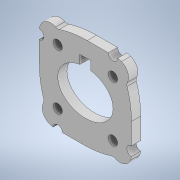
# Autodesk Inventor part: Część18
Saved by Autodesk Inventor 2021 (Build 250183000, 183)
## iProperties
Created: 2023-10-30
Part Number: Część18
Material: Ogólny
Document SubType Name: Modeling
Designer: Jakub
Density: 1 g/cm^3
Appearance: Domyślna
Author: Jakub
Autodesk Inventor part; units mm, degrees
ref_plane "YZ Plane" through (0, 0, 0) normal (1, 0, 0) x (0, 1, 0)
ref_plane "XZ Plane" through (0, 0, 0) normal (0, 1, 0) x (-1, 0, 0)
ref_plane "XY Plane" through (0, 0, 0) normal (0, 0, 1) x (1, 0, 0)
sketch "Szkic1" plane through (0, 0, 0) normal (0, 0, 1) x (1, 0, 0)
  line L0 (0, 0) -> (25, 0)
  line L1 (25, 0) -> (25, 16.5)
  line L2 (16.5, 25) -> (0, 25)
  line L3 (0, 25) -> (0, 0)
  line L4 (0, 0) -> (-25, 0)
  line L5 (-25, 0) -> (-25, -16.5)
  line L6 (-16.5, -25) -> (0, -25)
  line L7 (0, -25) -> (0, 0)
  line L8 (0, 0) -> (-25, 0)
  line L9 (-25, 0) -> (-25, 16.5)
  line L10 (-16.5, 25) -> (0, 25)
  line L11 (0, 25) -> (0, 0)
  line L12 (0, 0) -> (25, 0)
  line L13 (25, 0) -> (25, -16.5)
  line L14 (16.5, -25) -> (0, -25)
  line L15 (0, -25) -> (0, 0)
  line L16 (0, 0) -> (0, -12)
  line L17 (0, -12) -> (0, 0)
  line L18 (0, 0) -> (-15, 0)
  line L19 (-15, 0) -> (15, 0)
  line L20 (15, 0) -> (15, 12)
  line L21 (15, 12) -> (-15, 12)
  line L22 (-15, 12) -> (-15, -0.7896)
  line L23 (-15, -0.7896) -> (-15, -12)
  line L24 (-15, -12) -> (0, -12)
  line L25 (15, -12) -> (15, 0)
  line L26 (15, -12) -> (0, -12)
  ellipse E0 centre (0, 0) end of major axis (-15, 0) minor radius 12
  line L27 (0, 0) -> (0, 16.5)
  line L28 (0, 16.5) -> (3, 16.5)
  line L29 (3, 16.5) -> (3, 11.7576)
  line L30 (0, 16.5) -> (-3, 16.5)
  line L31 (-3, 16.5) -> (-3, 11.7576)
  arc A0 (-16.5, 25) -> (-25, 16.5) centre (-16.5, 16.5) ccw
  arc A1 (25, 16.5) -> (16.5, 25) centre (16.5, 16.5) ccw
  arc A2 (16.5, -25) -> (25, -16.5) centre (16.5, -16.5) ccw
  arc A3 (-25, -16.5) -> (-16.5, -25) centre (-16.5, -16.5) ccw
  point P0 (25, 25)
  point P1 (-25, -25)
  point P2 (-25, 25)
  point P3 (25, -25)
  dimension "d0" = 25
  dimension "d1" = 25
  dimension "d2" = 25
  dimension "d3" = 25
  dimension "d4" = 12
  dimension "d5" = 15
  dimension "d6" = 30
  dimension "d7" = 12
  dimension "d8" = 16.5
  dimension "d9" = 3
  dimension "d10" = 3
  dimension "d11" = 8.5
  constraints: 64 end point, 20 point on line, 12 perpendicular, 8 parallel, 8 point on circle, 8 tangent, 4 centre point, 4 horizontal, 3 equal radius, 3 vertical, 1 coincident, 5 other
  measures "d0" distance of L2.end point (25, 25)
  measures "d1" distance of point (25, 25) L0.end
  measures "d2" distance of L6.end point (-25, -25)
  measures "d3" distance of point (-25, -25) L4.end
  measures "d4" distance of L0.start L16.end
  measures "d5" distance of L0.start L18.end
  measures "d6" distance of L18.end L19.end
  measures "d7" distance of L19.end L20.end
  measures "d8" distance of L27.start L27.end
  measures "d9" distance of L27.end L28.end
  measures "d10" distance of L27.end L30.end
  measures "d11" radius of A0
extrude "Wyciągnięcie proste1" add sketch "Szkic1" along normal blind 5 contours L20 L21 L29 L28 L3 L2 A1 L1 L0 | E0 L29 L21 L20 | L0 L13 A2 L14 L7 L26 L25 | L25 L26 E0 | L22 L23 L24 L7 L6 A3 L5 L4 | L4 L9 A0 L10 L3 L30 L31 L21 L22 | E0 L24 L23 L22 | L22 L21 L31 E0
sketch "Szkic2" plane through (0, 0, 5) normal (0, 0, 1) x (1, 0, 0)
  line L0 (-25, 16.5) -> (-25, -16.5) projected
  line L1 (-25, 0) -> (-15, 0)
  ellipse E0 centre (0, 0) end of major axis (15, 0) minor radius 12 (-3, 11.7576) -> (3, 11.7576) ccw projected
  line L2 (-15, 0) -> (-15, 25)
  line L3 (16.5, 25) -> (-16.5, 25) projected
  line L4 (-15, 0) -> (-15, -25)
  line L5 (-16.5, -25) -> (16.5, -25) projected
  line L6 (15, 0) -> (15, -25)
  line L7 (15, 0) -> (15, 25)
  line L8 (-15, 25) -> (-15, 15)
  line L9 (-15, 15) -> (25, 15)
  line L10 (25, -16.5) -> (25, 16.5) projected
  line L11 (-15, 15) -> (-25, 15)
  line L12 (-15, -25) -> (-15, -15)
  line L13 (-15, -15) -> (-25, -15)
  line L14 (-15, -15) -> (25, -15)
  circle A0 centre (-15, 15) radius 2.5
  circle A1 centre (15, 15) radius 2.5
  circle A2 centre (15, -15) radius 2.5
  circle A3 centre (-15, -15) radius 2.5
  circle A4 centre (25, 15) radius 2.5
  circle A5 centre (25, -15) radius 2.5
  circle A6 centre (15, -25) radius 2.5
  circle A7 centre (-15, -25) radius 2.5
  circle A8 centre (-25, -15) radius 2.5
  circle A9 centre (-25, 15) radius 2.5
  circle A10 centre (-15, 25) radius 2.5
  circle A11 centre (15, 25) radius 2.5
  dimension "d14" = 10
  dimension "d15" = 10
  dimension "d16" = 5
  dimension "d17" = 5
  dimension "d18" = 5
  dimension "d19" = 5
  dimension "d20" = 5
  dimension "d21" = 5
  dimension "d22" = 5
  dimension "d23" = 5
  dimension "d24" = 5
  dimension "d25" = 5
  dimension "d26" = 5
  dimension "d27" = 5
  constraints: 22 end point, 17 point on line, 12 centre point, 10 coincident, 4 perpendicular, 1 horizontal, 1 midpoint, 1 vertical, 3 other
  measures "d14" distance of L2.end L8.end
  measures "d15" distance of L4.end L12.end
  measures "d16" diameter of A0
  measures "d17" diameter of A1
  measures "d18" diameter of A2
  measures "d19" diameter of A3
  measures "d20" diameter of A4
  measures "d21" diameter of A5
  measures "d22" diameter of A6
  measures "d23" diameter of A7
  measures "d24" diameter of A8
  measures "d25" diameter of A9
  measures "d26" diameter of A10
  measures "d27" diameter of A11
extrude "Wyciągnięcie proste2" cut sketch "Szkic2" against normal blind 5 contours L11 A9 L0 | L0 A9 L11 | A0 L2 L11 | L11 L2 A0 | A8 L13 L0 | L0 L13 A8 | L9 A0 L2 | L2 A0 L9 | A3 L14 L4 | L4 L13 A3 | A10 L3 L2 | L2 L3 A10 | L13 L4 A3 | A2 L14 L6 | L6 L14 A2 | A1 L9 L7 | L7 L9 A1 | L14 A3 L4 | A1 L7 L9 | L14 A2 L6 | L6 A2 L14 | L7 A1 L9 | A11 L7 L3 | L3 L7 A11 | A7 L5 L4 | L4 L5 A7 | A5 L10 L14 | L14 L10 A5 | A4 L10 L9 | L9 L10 A4 | A6 L5 L6 | L6 L5 A6
fillet "Zaokrąglenie1" radius 6 4 edges at (24.9411, 17.4993, 2.5) (17.4993, -24.9411, 2.5) (-24.9411, -17.4993, 2.5) (-17.4993, 24.9411, 2.5)
fillet "Zaokrąglenie2" radius 50 4 edges at (-12.5, 25, 2.5) (-25, -12.5, 2.5) (12.5, -25, 2.5) (25, 12.5, 2.5)
equation "\"d28\" = d17"
